Autodesk Fusion 360 part; units mm, degrees
(part 2 of 3)
sketch "Schizzo3 (7)" plane through (0, 0, 39.9) normal (0, 0, 1) x (1, 0, 0) in component "03A_Fermaglio_anti_sollevamento_Est_M3"
  line L0 (48.5, -5) -> (55, -5)
  line L1 (55, -5) -> (55, 5)
  line L2 (55, 5) -> (48.5, 5)
  line L3 (48.5, 5) -> (48.5, -5)
extrude "Estrusione_Linguetta_fermaglio_Est" add sketch "Schizzo3 (7)" along normal blind 3 bodies 8 in component "03A_Fermaglio_anti_sollevamento_Est_M3"
sketch "Schizzo4 (7)" plane through (0, 0, 33) normal (0, 0, 1) x (1, 0, 0) in component "03A_Fermaglio_anti_sollevamento_Est_M3"
  circle A0 centre (58.5, 0) radius 1.6
extrude "Foro_M3_fermaglio_Est" cut sketch "Schizzo4 (7)" along normal blind 3 bodies 8 in component "03A_Fermaglio_anti_sollevamento_Est_M3"
ref_plane "Piano di lavoro1" through (0, 0, 33) normal (0, 0, 1) x (1, 0, 0) in component "03A_Fermaglio_anti_sollevamento_Ovest_M3"
ref_plane "Piano di lavoro2" through (0, 0, 36) normal (0, 0, 1) x (1, 0, 0) in component "03A_Fermaglio_anti_sollevamento_Ovest_M3"
ref_plane "Piano di lavoro3" through (0, 0, 39.9) normal (0, 0, 1) x (1, 0, 0) in component "03A_Fermaglio_anti_sollevamento_Ovest_M3"
sketch "Schizzo1 (10)" plane through (0, 0, 33) normal (0, 0, 1) x (1, 0, 0) in component "03A_Fermaglio_anti_sollevamento_Ovest_M3"
  line L0 (-61.5, -5) -> (-51.5, -5)
  line L1 (-51.5, -5) -> (-51.5, 5)
  line L2 (-51.5, 5) -> (-61.5, 5)
  line L3 (-61.5, 5) -> (-61.5, -5)
extrude "Estrusione_Piede_fermaglio_Ovest" add sketch "Schizzo1 (10)" along normal blind 3 separate body makes body 9 in component "03A_Fermaglio_anti_sollevamento_Ovest_M3"
sketch "Schizzo2 (8)" plane through (0, 0, 36) normal (0, 0, 1) x (1, 0, 0) in component "03A_Fermaglio_anti_sollevamento_Ovest_M3"
  line L0 (-55, -5) -> (-52, -5)
  line L1 (-52, -5) -> (-52, 5)
  line L2 (-52, 5) -> (-55, 5)
  line L3 (-55, 5) -> (-55, -5)
extrude "Estrusione_Montante_fermaglio_Ovest" add sketch "Schizzo2 (8)" along normal blind 3.9 bodies 9 in component "03A_Fermaglio_anti_sollevamento_Ovest_M3"
sketch "Schizzo3 (8)" plane through (0, 0, 39.9) normal (0, 0, 1) x (1, 0, 0) in component "03A_Fermaglio_anti_sollevamento_Ovest_M3"
  line L0 (-55, -5) -> (-48.5, -5)
  line L1 (-48.5, -5) -> (-48.5, 5)
  line L2 (-48.5, 5) -> (-55, 5)
  line L3 (-55, 5) -> (-55, -5)
extrude "Estrusione_Linguetta_fermaglio_Ovest" add sketch "Schizzo3 (8)" along normal blind 3 bodies 9 in component "03A_Fermaglio_anti_sollevamento_Ovest_M3"
sketch "Schizzo4 (8)" plane through (0, 0, 33) normal (0, 0, 1) x (1, 0, 0) in component "03A_Fermaglio_anti_sollevamento_Ovest_M3"
  circle A0 centre (-58.5, 0) radius 1.6
extrude "Foro_M3_fermaglio_Ovest" cut sketch "Schizzo4 (8)" along normal blind 3 bodies 9 in component "03A_Fermaglio_anti_sollevamento_Ovest_M3"
ref_plane "Piano di lavoro1" through (0, 0, 33) normal (0, 0, 1) x (1, 0, 0) in component "03A_Fermaglio_anti_sollevamento_Nord_M3"
ref_plane "Piano di lavoro2" through (0, 0, 36) normal (0, 0, 1) x (1, 0, 0) in component "03A_Fermaglio_anti_sollevamento_Nord_M3"
ref_plane "Piano di lavoro3" through (0, 0, 39.9) normal (0, 0, 1) x (1, 0, 0) in component "03A_Fermaglio_anti_sollevamento_Nord_M3"
sketch "Schizzo1 (11)" plane through (0, 0, 33) normal (0, 0, 1) x (1, 0, 0) in component "03A_Fermaglio_anti_sollevamento_Nord_M3"
  line L0 (-5, 51.5) -> (5, 51.5)
  line L1 (5, 51.5) -> (5, 61.5)
  line L2 (5, 61.5) -> (-5, 61.5)
  line L3 (-5, 61.5) -> (-5, 51.5)
extrude "Estrusione_Piede_fermaglio_Nord" add sketch "Schizzo1 (11)" along normal blind 3 separate body makes body 10 in component "03A_Fermaglio_anti_sollevamento_Nord_M3"
sketch "Schizzo2 (9)" plane through (0, 0, 36) normal (0, 0, 1) x (1, 0, 0) in component "03A_Fermaglio_anti_sollevamento_Nord_M3"
  line L0 (-5, 52) -> (5, 52)
  line L1 (5, 52) -> (5, 55)
  line L2 (5, 55) -> (-5, 55)
  line L3 (-5, 55) -> (-5, 52)
extrude "Estrusione_Montante_fermaglio_Nord" add sketch "Schizzo2 (9)" along normal blind 3.9 bodies 10 in component "03A_Fermaglio_anti_sollevamento_Nord_M3"
sketch "Schizzo3 (9)" plane through (0, 0, 39.9) normal (0, 0, 1) x (1, 0, 0) in component "03A_Fermaglio_anti_sollevamento_Nord_M3"
  line L0 (-5, 48.5) -> (5, 48.5)
  line L1 (5, 48.5) -> (5, 55)
  line L2 (5, 55) -> (-5, 55)
  line L3 (-5, 55) -> (-5, 48.5)
extrude "Estrusione_Linguetta_fermaglio_Nord" add sketch "Schizzo3 (9)" along normal blind 3 bodies 10 in component "03A_Fermaglio_anti_sollevamento_Nord_M3"
sketch "Schizzo4 (9)" plane through (0, 0, 33) normal (0, 0, 1) x (1, 0, 0) in component "03A_Fermaglio_anti_sollevamento_Nord_M3"
  circle A0 centre (0, 58.5) radius 1.6
extrude "Foro_M3_fermaglio_Nord" cut sketch "Schizzo4 (9)" along normal blind 3 bodies 10 in component "03A_Fermaglio_anti_sollevamento_Nord_M3"
ref_plane "Piano di lavoro1" through (0, 0, 33) normal (0, 0, 1) x (1, 0, 0) in component "03A_Fermaglio_anti_sollevamento_Sud_M3"
ref_plane "Piano di lavoro2" through (0, 0, 36) normal (0, 0, 1) x (1, 0, 0) in component "03A_Fermaglio_anti_sollevamento_Sud_M3"
ref_plane "Piano di lavoro3" through (0, 0, 39.9) normal (0, 0, 1) x (1, 0, 0) in component "03A_Fermaglio_anti_sollevamento_Sud_M3"
sketch "Schizzo1 (12)" plane through (0, 0, 33) normal (0, 0, 1) x (1, 0, 0) in component "03A_Fermaglio_anti_sollevamento_Sud_M3"
  line L0 (-5, -61.5) -> (5, -61.5)
  line L1 (5, -61.5) -> (5, -51.5)
  line L2 (5, -51.5) -> (-5, -51.5)
  line L3 (-5, -51.5) -> (-5, -61.5)
extrude "Estrusione_Piede_fermaglio_Sud" add sketch "Schizzo1 (12)" along normal blind 3 separate body makes body 11 in component "03A_Fermaglio_anti_sollevamento_Sud_M3"
sketch "Schizzo2 (10)" plane through (0, 0, 36) normal (0, 0, 1) x (1, 0, 0) in component "03A_Fermaglio_anti_sollevamento_Sud_M3"
  line L0 (-5, -55) -> (5, -55)
  line L1 (5, -55) -> (5, -52)
  line L2 (5, -52) -> (-5, -52)
  line L3 (-5, -52) -> (-5, -55)
extrude "Estrusione_Montante_fermaglio_Sud" add sketch "Schizzo2 (10)" along normal blind 3.9 bodies 11 in component "03A_Fermaglio_anti_sollevamento_Sud_M3"
sketch "Schizzo3 (10)" plane through (0, 0, 39.9) normal (0, 0, 1) x (1, 0, 0) in component "03A_Fermaglio_anti_sollevamento_Sud_M3"
  line L0 (-5, -55) -> (5, -55)
  line L1 (5, -55) -> (5, -48.5)
  line L2 (5, -48.5) -> (-5, -48.5)
  line L3 (-5, -48.5) -> (-5, -55)
extrude "Estrusione_Linguetta_fermaglio_Sud" add sketch "Schizzo3 (10)" along normal blind 3 bodies 11 in component "03A_Fermaglio_anti_sollevamento_Sud_M3"
sketch "Schizzo4 (10)" plane through (0, 0, 33) normal (0, 0, 1) x (1, 0, 0) in component "03A_Fermaglio_anti_sollevamento_Sud_M3"
  circle A0 centre (0, -58.5) radius 1.6
extrude "Foro_M3_fermaglio_Sud" cut sketch "Schizzo4 (10)" along normal blind 3 bodies 11 in component "03A_Fermaglio_anti_sollevamento_Sud_M3"
ref_plane "Piano di lavoro1" through (0, 0, 45.5) normal (0, 0, 1) x (1, 0, 0) in component "04_Torretta_parte_fissa_azimut"
sketch "Schizzo1 (13)" plane through (0, 0, 45.5) normal (0, 0, 1) x (1, 0, 0) in component "04_Torretta_parte_fissa_azimut"
  line L0 (-40, -35) -> (40, -35)
  line L1 (40, -35) -> (40, 35)
  line L2 (40, 35) -> (-40, 35)
  line L3 (-40, 35) -> (-40, -35)
extrude "Estrusione_Base_parte_fissa" add sketch "Schizzo1 (13)" along normal blind 4 separate body makes body 12 in component "04_Torretta_parte_fissa_azimut"
ref_plane "Piano di lavoro2" through (0, 0, 39.5) normal (0, 0, 1) x (1, 0, 0) in component "04_Torretta_parte_fissa_azimut"
sketch "Schizzo2 (11)" plane through (0, 0, 39.5) normal (0, 0, 1) x (1, 0, 0) in component "04_Torretta_parte_fissa_azimut"
  circle A0 centre (-19, 0) radius 5
extrude "Estrusione_Distanziale_telaio_M3_01" add sketch "Schizzo2 (11)" along normal blind 6.2 bodies 12 in component "04_Torretta_parte_fissa_azimut"
sketch "Schizzo3 (11)" plane through (0, 0, 39.5) normal (0, 0, 1) x (1, 0, 0) in component "04_Torretta_parte_fissa_azimut"
  circle A0 centre (-19, 0) radius 1.6
extrude "Foro_M3_base_fissa_01" cut sketch "Schizzo3 (11)" along normal blind 10 bodies 12 in component "04_Torretta_parte_fissa_azimut"
sketch "Schizzo4 (11)" plane through (0, 0, 39.5) normal (0, 0, 1) x (1, 0, 0) in component "04_Torretta_parte_fissa_azimut"
  circle A0 centre (19, 0) radius 5
extrude "Estrusione_Distanziale_telaio_M3_02" add sketch "Schizzo4 (11)" along normal blind 6.2 bodies 12 in component "04_Torretta_parte_fissa_azimut"
sketch "Schizzo5 (6)" plane through (0, 0, 39.5) normal (0, 0, 1) x (1, 0, 0) in component "04_Torretta_parte_fissa_azimut"
  circle A0 centre (19, 0) radius 1.6
extrude "Foro_M3_base_fissa_02" cut sketch "Schizzo5 (6)" along normal blind 10 bodies 12 in component "04_Torretta_parte_fissa_azimut"
sketch "Schizzo6 (6)" plane through (0, 0, 39.5) normal (0, 0, 1) x (1, 0, 0) in component "04_Torretta_parte_fissa_azimut"
  circle A0 centre (0, -19) radius 5
extrude "Estrusione_Distanziale_telaio_M3_03" add sketch "Schizzo6 (6)" along normal blind 6.2 bodies 12 in component "04_Torretta_parte_fissa_azimut"
sketch "Schizzo7 (6)" plane through (0, 0, 39.5) normal (0, 0, 1) x (1, 0, 0) in component "04_Torretta_parte_fissa_azimut"
  circle A0 centre (0, -19) radius 1.6
extrude "Foro_M3_base_fissa_03" cut sketch "Schizzo7 (6)" along normal blind 10 bodies 12 in component "04_Torretta_parte_fissa_azimut"
sketch "Schizzo8 (6)" plane through (0, 0, 39.5) normal (0, 0, 1) x (1, 0, 0) in component "04_Torretta_parte_fissa_azimut"
  circle A0 centre (0, 19) radius 5
extrude "Estrusione_Distanziale_telaio_M3_04" add sketch "Schizzo8 (6)" along normal blind 6.2 bodies 12 in component "04_Torretta_parte_fissa_azimut"
sketch "Schizzo9 (6)" plane through (0, 0, 39.5) normal (0, 0, 1) x (1, 0, 0) in component "04_Torretta_parte_fissa_azimut"
  circle A0 centre (0, 19) radius 1.6
extrude "Foro_M3_base_fissa_04" cut sketch "Schizzo9 (6)" along normal blind 10 bodies 12 in component "04_Torretta_parte_fissa_azimut"
sketch "Schizzo10 (6)" plane through (0, 0, 45.5) normal (0, 0, 1) x (1, 0, 0) in component "04_Torretta_parte_fissa_azimut"
  line L0 (19.0919, 14.1421) -> (25.4558, 20.5061)
  line L1 (25.4558, 20.5061) -> (20.5061, 25.4558)
  line L2 (20.5061, 25.4558) -> (14.1421, 19.0919)
  line L3 (14.1421, 19.0919) -> (19.0919, 14.1421)
extrude "Passaggio_9x7_comune_servi_cannone_base_fissa" cut sketch "Schizzo10 (6)" along normal blind 4 bodies 12 in component "04_Torretta_parte_fissa_azimut"
sketch "Schizzo11 (6)" plane through (0, 0, 45.5) normal (0, 0, 1) x (1, 0, 0) in component "04_Torretta_parte_fissa_azimut"
  line L0 (-30.5, -19.5) -> (-25.5, -19.5)
  line L1 (-25.5, -19.5) -> (-25.5, -17.5)
  line L2 (-25.5, -17.5) -> (-30.5, -17.5)
  line L3 (-30.5, -17.5) -> (-30.5, -19.5)
extrude "Asola_fermacavo_Servo_sinistro_01" cut sketch "Schizzo11 (6)" along normal blind 4 bodies 12 in component "04_Torretta_parte_fissa_azimut"
sketch "Schizzo12 (5)" plane through (0, 0, 45.5) normal (0, 0, 1) x (1, 0, 0) in component "04_Torretta_parte_fissa_azimut"
  line L0 (-30.5, -12.5) -> (-25.5, -12.5)
  line L1 (-25.5, -12.5) -> (-25.5, -10.5)
  line L2 (-25.5, -10.5) -> (-30.5, -10.5)
  line L3 (-30.5, -10.5) -> (-30.5, -12.5)
extrude "Asola_fermacavo_Servo_sinistro_02" cut sketch "Schizzo12 (5)" along normal blind 4 bodies 12 in component "04_Torretta_parte_fissa_azimut"
sketch "Schizzo13 (5)" plane through (0, 0, 45.5) normal (0, 0, 1) x (1, 0, 0) in component "04_Torretta_parte_fissa_azimut"
  line L0 (-2.5, -11.5) -> (2.5, -11.5)
  line L1 (2.5, -11.5) -> (2.5, -9.5)
  line L2 (2.5, -9.5) -> (-2.5, -9.5)
  line L3 (-2.5, -9.5) -> (-2.5, -11.5)
extrude "Asola_fermacavo_Cannone_01" cut sketch "Schizzo13 (5)" along normal blind 4 bodies 12 in component "04_Torretta_parte_fissa_azimut"
sketch "Schizzo14 (4)" plane through (0, 0, 45.5) normal (0, 0, 1) x (1, 0, 0) in component "04_Torretta_parte_fissa_azimut"
  line L0 (-2.5, -4.5) -> (2.5, -4.5)
  line L1 (2.5, -4.5) -> (2.5, -2.5)
  line L2 (2.5, -2.5) -> (-2.5, -2.5)
  line L3 (-2.5, -2.5) -> (-2.5, -4.5)
extrude "Asola_fermacavo_Cannone_02" cut sketch "Schizzo14 (4)" along normal blind 4 bodies 12 in component "04_Torretta_parte_fissa_azimut"
sketch "Schizzo15 (4)" plane through (0, 0, 45.5) normal (0, 0, 1) x (1, 0, 0) in component "04_Torretta_parte_fissa_azimut"
  line L0 (25.5, -19.5) -> (30.5, -19.5)
  line L1 (30.5, -19.5) -> (30.5, -17.5)
  line L2 (30.5, -17.5) -> (25.5, -17.5)
  line L3 (25.5, -17.5) -> (25.5, -19.5)
extrude "Asola_fermacavo_Servo_destro_01" cut sketch "Schizzo15 (4)" along normal blind 4 bodies 12 in component "04_Torretta_parte_fissa_azimut"
sketch "Schizzo16 (4)" plane through (0, 0, 45.5) normal (0, 0, 1) x (1, 0, 0) in component "04_Torretta_parte_fissa_azimut"
  line L0 (25.5, -12.5) -> (30.5, -12.5)
  line L1 (30.5, -12.5) -> (30.5, -10.5)
  line L2 (30.5, -10.5) -> (25.5, -10.5)
  line L3 (25.5, -10.5) -> (25.5, -12.5)
extrude "Asola_fermacavo_Servo_destro_02" cut sketch "Schizzo16 (4)" along normal blind 4 bodies 12 in component "04_Torretta_parte_fissa_azimut"
ref_plane "Piano di lavoro3" through (-40, 0, 0) normal (1, 0, 0) x (0, 1, 0) in component "04_Torretta_parte_fissa_azimut"
sketch "Schizzo17 (4)" plane through (-40, 0, 0) normal (1, 0, 0) x (0, 0, -1) in component "04_Torretta_parte_fissa_azimut"
  line L0 (-49.5, -35) -> (-99.5, -35)
  line L1 (-99.5, -35) -> (-99.5, 35)
  line L2 (-99.5, 35) -> (-49.5, 35)
  line L3 (-49.5, 35) -> (-49.5, -35)
extrude "Estrusione_Parete_fissa_Sinistra" add sketch "Schizzo17 (4)" along normal blind 4 bodies 12 in component "04_Torretta_parte_fissa_azimut"
ref_plane "Piano di lavoro4" through (-40, 0, 0) normal (1, 0, 0) x (0, 1, 0) in component "04_Torretta_parte_fissa_azimut"
sketch "Schizzo18 (4)" plane through (-40, 0, 0) normal (1, 0, 0) x (0, 0, -1) in component "04_Torretta_parte_fissa_azimut"
  line L0 (-74.9, -17.5) -> (-88.1, -17.5)
  line L1 (-88.1, -17.5) -> (-88.1, 6.2)
  line L2 (-88.1, 6.2) -> (-74.9, 6.2)
  line L3 (-74.9, 6.2) -> (-74.9, -17.5)
extrude "Finestra_inserimento_SG90_Sinistra" cut sketch "Schizzo18 (4)" along normal blind 4 bodies 12 in component "04_Torretta_parte_fissa_azimut"
ref_plane "Piano di lavoro5" through (-40, 0, 0) normal (1, 0, 0) x (0, 1, 0) in component "04_Torretta_parte_fissa_azimut"
sketch "Schizzo19 (3)" plane through (-40, 0, 0) normal (1, 0, 0) x (0, 0, -1) in component "04_Torretta_parte_fissa_azimut"
  line L0 (-70.4, -8.15) -> (-74.9, -8.15)
  line L1 (-74.9, -8.15) -> (-74.9, -3.15)
  line L2 (-74.9, -3.15) -> (-70.4, -3.15)
  line L3 (-70.4, -3.15) -> (-70.4, -8.15)
extrude "Diramazione_cavo_5x4_5_SG90_Sinistra" cut sketch "Schizzo19 (3)" along normal blind 4 bodies 12 in component "04_Torretta_parte_fissa_azimut"
ref_plane "Piano di lavoro6" through (36, 0, 0) normal (1, 0, 0) x (0, 1, 0) in component "04_Torretta_parte_fissa_azimut"
sketch "Schizzo20 (3)" plane through (36, 0, 0) normal (1, 0, 0) x (0, 0, -1) in component "04_Torretta_parte_fissa_azimut"
  line L0 (-49.5, -35) -> (-99.5, -35)
  line L1 (-99.5, -35) -> (-99.5, 35)
  line L2 (-99.5, 35) -> (-49.5, 35)
  line L3 (-49.5, 35) -> (-49.5, -35)
extrude "Estrusione_Parete_fissa_Destra" add sketch "Schizzo20 (3)" along normal blind 4 bodies 12 in component "04_Torretta_parte_fissa_azimut"
ref_plane "Piano di lavoro7" through (36, 0, 0) normal (1, 0, 0) x (0, 1, 0) in component "04_Torretta_parte_fissa_azimut"
sketch "Schizzo21 (3)" plane through (36, 0, 0) normal (1, 0, 0) x (0, 0, -1) in component "04_Torretta_parte_fissa_azimut"
  line L0 (-74.9, -17.5) -> (-88.1, -17.5)
  line L1 (-88.1, -17.5) -> (-88.1, 6.2)
  line L2 (-88.1, 6.2) -> (-74.9, 6.2)
  line L3 (-74.9, 6.2) -> (-74.9, -17.5)
extrude "Finestra_inserimento_SG90_Destra" cut sketch "Schizzo21 (3)" along normal blind 4 bodies 12 in component "04_Torretta_parte_fissa_azimut"
ref_plane "Piano di lavoro8" through (36, 0, 0) normal (1, 0, 0) x (0, 1, 0) in component "04_Torretta_parte_fissa_azimut"
sketch "Schizzo22 (3)" plane through (36, 0, 0) normal (1, 0, 0) x (0, 0, -1) in component "04_Torretta_parte_fissa_azimut"
  line L0 (-70.4, -8.15) -> (-74.9, -8.15)
  line L1 (-74.9, -8.15) -> (-74.9, -3.15)
  line L2 (-74.9, -3.15) -> (-70.4, -3.15)
  line L3 (-70.4, -3.15) -> (-70.4, -8.15)
extrude "Diramazione_cavo_5x4_5_SG90_Destra" cut sketch "Schizzo22 (3)" along normal blind 4 bodies 12 in component "04_Torretta_parte_fissa_azimut"
ref_plane "Piano di lavoro9" through (0, 0, 72.4) normal (0, 0, 1) x (1, 0, 0) in component "04_Torretta_parte_fissa_azimut"
sketch "Schizzo23 (2)" plane through (0, 0, 72.4) normal (0, 0, 1) x (1, 0, 0) in component "04_Torretta_parte_fissa_azimut"
  line L0 (-63.5, -24.8) -> (-40, -24.8)
  line L1 (-40, -24.8) -> (-40, 13.5)
  line L2 (-40, 13.5) -> (-63.5, 13.5)
  line L3 (-63.5, 13.5) -> (-63.5, -24.8)
extrude "Estrusione_Slitta_SG90_Sinistra_ripiano_Inferiore" add sketch "Schizzo23 (2)" along normal blind 2.5 bodies 12 in component "04_Torretta_parte_fissa_azimut"
ref_plane "Piano di lavoro10" through (0, 0, 88.1) normal (0, 0, 1) x (1, 0, 0) in component "04_Torretta_parte_fissa_azimut"
sketch "Schizzo24 (2)" plane through (0, 0, 88.1) normal (0, 0, 1) x (1, 0, 0) in component "04_Torretta_parte_fissa_azimut"
  line L0 (-63.5, -24.8) -> (-40, -24.8)
  line L1 (-40, -24.8) -> (-40, 13.5)
  line L2 (-40, 13.5) -> (-63.5, 13.5)
  line L3 (-63.5, 13.5) -> (-63.5, -24.8)
extrude "Estrusione_Slitta_SG90_Sinistra_ripiano_Superiore" add sketch "Schizzo24 (2)" along normal blind 2.5 bodies 12 in component "04_Torretta_parte_fissa_azimut"
ref_plane "Piano di lavoro11" through (0, 0, 72.4) normal (0, 0, 1) x (1, 0, 0) in component "04_Torretta_parte_fissa_azimut"
sketch "Schizzo25 (2)" plane through (0, 0, 72.4) normal (0, 0, 1) x (1, 0, 0) in component "04_Torretta_parte_fissa_azimut"
  line L0 (-63.5, -8.15) -> (-61.5, -8.15)
  line L1 (-61.5, -8.15) -> (-61.5, -3.15)
  line L2 (-61.5, -3.15) -> (-63.5, -3.15)
  line L3 (-63.5, -3.15) -> (-63.5, -8.15)
extrude "Uscita_cavo_5x2_SG90_Sinistra" cut sketch "Schizzo25 (2)" along normal blind 2.5 bodies 12 in component "04_Torretta_parte_fissa_azimut"
ref_plane "Piano di lavoro12" through (-63.5, 0, 0) normal (1, 0, 0) x (0, 1, 0) in component "04_Torretta_parte_fissa_azimut"
sketch "Schizzo26 (2)" plane through (-63.5, 0, 0) normal (1, 0, 0) x (0, 0, -1) in component "04_Torretta_parte_fissa_azimut"
  line L0 (-74.9, -24.8) -> (-88.1, -24.8)
  line L1 (-88.1, -24.8) -> (-88.1, -22.3)
  line L2 (-88.1, -22.3) -> (-74.9, -22.3)
  line L3 (-74.9, -22.3) -> (-74.9, -24.8)
extrude "Estrusione_Slitta_SG90_Sinistra_guida_01" add sketch "Schizzo26 (2)" along normal blind 23.5 bodies 12 in component "04_Torretta_parte_fissa_azimut"
ref_plane "Piano di lavoro13" through (-63.5, 0, 0) normal (1, 0, 0) x (0, 1, 0) in component "04_Torretta_parte_fissa_azimut"
sketch "Schizzo27 (2)" plane through (-63.5, 0, 0) normal (1, 0, 0) x (0, 0, -1) in component "04_Torretta_parte_fissa_azimut"
  line L0 (-74.9, 11) -> (-88.1, 11)
  line L1 (-88.1, 11) -> (-88.1, 13.5)
  line L2 (-88.1, 13.5) -> (-74.9, 13.5)
  line L3 (-74.9, 13.5) -> (-74.9, 11)
extrude "Estrusione_Slitta_SG90_Sinistra_guida_02" add sketch "Schizzo27 (2)" along normal blind 23.5 bodies 12 in component "04_Torretta_parte_fissa_azimut"
ref_plane "Piano di lavoro14" through (-63.5, 0, 0) normal (1, 0, 0) x (0, 1, 0) in component "04_Torretta_parte_fissa_azimut"
sketch "Schizzo28 (2)" plane through (-63.5, 0, 0) normal (1, 0, 0) x (0, 0, -1) in component "04_Torretta_parte_fissa_azimut"
  circle A0 centre (-81.5, -23.55) radius 1.1
extrude "Preforo_M2_5_slitta_Sinistra_01" cut sketch "Schizzo28 (2)" along normal blind 23.5 bodies 12 in component "04_Torretta_parte_fissa_azimut"
ref_plane "Piano di lavoro15" through (-63.5, 0, 0) normal (1, 0, 0) x (0, 1, 0) in component "04_Torretta_parte_fissa_azimut"
sketch "Schizzo29 (2)" plane through (-63.5, 0, 0) normal (1, 0, 0) x (0, 0, -1) in component "04_Torretta_parte_fissa_azimut"
  circle A0 centre (-81.5, 12.25) radius 1.1
extrude "Preforo_M2_5_slitta_Sinistra_02" cut sketch "Schizzo29 (2)" along normal blind 23.5 bodies 12 in component "04_Torretta_parte_fissa_azimut"
ref_plane "Piano di lavoro16" through (0, 0, 72.4) normal (0, 0, 1) x (1, 0, 0) in component "04_Torretta_parte_fissa_azimut"
sketch "Schizzo30 (2)" plane through (0, 0, 72.4) normal (0, 0, 1) x (1, 0, 0) in component "04_Torretta_parte_fissa_azimut"
  line L0 (40, -24.8) -> (63.5, -24.8)
  line L1 (63.5, -24.8) -> (63.5, 13.5)
  line L2 (63.5, 13.5) -> (40, 13.5)
  line L3 (40, 13.5) -> (40, -24.8)
extrude "Estrusione_Slitta_SG90_Destra_ripiano_Inferiore" add sketch "Schizzo30 (2)" along normal blind 2.5 bodies 12 in component "04_Torretta_parte_fissa_azimut"
ref_plane "Piano di lavoro17" through (0, 0, 88.1) normal (0, 0, 1) x (1, 0, 0) in component "04_Torretta_parte_fissa_azimut"
sketch "Schizzo31 (2)" plane through (0, 0, 88.1) normal (0, 0, 1) x (1, 0, 0) in component "04_Torretta_parte_fissa_azimut"
  line L0 (40, -24.8) -> (63.5, -24.8)
  line L1 (63.5, -24.8) -> (63.5, 13.5)
  line L2 (63.5, 13.5) -> (40, 13.5)
  line L3 (40, 13.5) -> (40, -24.8)
extrude "Estrusione_Slitta_SG90_Destra_ripiano_Superiore" add sketch "Schizzo31 (2)" along normal blind 2.5 bodies 12 in component "04_Torretta_parte_fissa_azimut"
ref_plane "Piano di lavoro18" through (0, 0, 72.4) normal (0, 0, 1) x (1, 0, 0) in component "04_Torretta_parte_fissa_azimut"
sketch "Schizzo32 (2)" plane through (0, 0, 72.4) normal (0, 0, 1) x (1, 0, 0) in component "04_Torretta_parte_fissa_azimut"
  line L0 (61.5, -8.15) -> (63.5, -8.15)
  line L1 (63.5, -8.15) -> (63.5, -3.15)
  line L2 (63.5, -3.15) -> (61.5, -3.15)
  line L3 (61.5, -3.15) -> (61.5, -8.15)
extrude "Uscita_cavo_5x2_SG90_Destra" cut sketch "Schizzo32 (2)" along normal blind 2.5 bodies 12 in component "04_Torretta_parte_fissa_azimut"
ref_plane "Piano di lavoro19" through (40, 0, 0) normal (1, 0, 0) x (0, 1, 0) in component "04_Torretta_parte_fissa_azimut"
sketch "Schizzo33 (2)" plane through (40, 0, 0) normal (1, 0, 0) x (0, 0, -1) in component "04_Torretta_parte_fissa_azimut"
  line L0 (-74.9, -24.8) -> (-88.1, -24.8)
  line L1 (-88.1, -24.8) -> (-88.1, -22.3)
  line L2 (-88.1, -22.3) -> (-74.9, -22.3)
  line L3 (-74.9, -22.3) -> (-74.9, -24.8)
extrude "Estrusione_Slitta_SG90_Destra_guida_01" add sketch "Schizzo33 (2)" along normal blind 23.5 bodies 12 in component "04_Torretta_parte_fissa_azimut"
ref_plane "Piano di lavoro20" through (40, 0, 0) normal (1, 0, 0) x (0, 1, 0) in component "04_Torretta_parte_fissa_azimut"
sketch "Schizzo34 (2)" plane through (40, 0, 0) normal (1, 0, 0) x (0, 0, -1) in component "04_Torretta_parte_fissa_azimut"
  line L0 (-74.9, 11) -> (-88.1, 11)
  line L1 (-88.1, 11) -> (-88.1, 13.5)
  line L2 (-88.1, 13.5) -> (-74.9, 13.5)
  line L3 (-74.9, 13.5) -> (-74.9, 11)
extrude "Estrusione_Slitta_SG90_Destra_guida_02" add sketch "Schizzo34 (2)" along normal blind 23.5 bodies 12 in component "04_Torretta_parte_fissa_azimut"
ref_plane "Piano di lavoro21" through (40, 0, 0) normal (1, 0, 0) x (0, 1, 0) in component "04_Torretta_parte_fissa_azimut"
sketch "Schizzo35 (2)" plane through (40, 0, 0) normal (1, 0, 0) x (0, 0, -1) in component "04_Torretta_parte_fissa_azimut"
  circle A0 centre (-81.5, -23.55) radius 1.1
extrude "Preforo_M2_5_slitta_Destra_01" cut sketch "Schizzo35 (2)" along normal blind 23.5 bodies 12 in component "04_Torretta_parte_fissa_azimut"
ref_plane "Piano di lavoro22" through (40, 0, 0) normal (1, 0, 0) x (0, 1, 0) in component "04_Torretta_parte_fissa_azimut"
sketch "Schizzo36 (2)" plane through (40, 0, 0) normal (1, 0, 0) x (0, 0, -1) in component "04_Torretta_parte_fissa_azimut"
  circle A0 centre (-81.5, 12.25) radius 1.1
extrude "Preforo_M2_5_slitta_Destra_02" cut sketch "Schizzo36 (2)" along normal blind 23.5 bodies 12 in component "04_Torretta_parte_fissa_azimut"
ref_plane "Piano di lavoro1" through (-63, 0, 0) normal (1, 0, 0) x (0, 1, 0) in component "05_Servo_TowerPro_SG90_Sinistro_riferimento"
sketch "Schizzo1 (14)" plane through (-63, 0, 0) normal (1, 0, 0) x (0, 0, -1) in component "05_Servo_TowerPro_SG90_Sinistro_riferimento"
  line L0 (-75.4, -17) -> (-87.6, -17)
  line L1 (-87.6, -17) -> (-87.6, 5.7)
  line L2 (-87.6, 5.7) -> (-75.4, 5.7)
  line L3 (-75.4, 5.7) -> (-75.4, -17)
extrude "Estrusione_Corpo_SG90_Sinistro" add sketch "Schizzo1 (14)" along normal blind 27 separate body makes body 13 in component "05_Servo_TowerPro_SG90_Sinistro_riferimento"
ref_plane "Piano di lavoro2" through (-36, 0, 0) normal (1, 0, 0) x (0, 1, 0) in component "05_Servo_TowerPro_SG90_Sinistro_riferimento"
sketch "Schizzo2 (12)" plane through (-36, 0, 0) normal (1, 0, 0) x (0, 0, -1) in component "05_Servo_TowerPro_SG90_Sinistro_riferimento"
  circle A0 centre (-81.5, 0) radius 3
extrude "Estrusione_Albero_uscita_SG90_Sinistro" add sketch "Schizzo2 (12)" along normal blind 3.3 bodies 13 in component "05_Servo_TowerPro_SG90_Sinistro_riferimento"
ref_plane "Piano di lavoro1" through (36, 0, 0) normal (1, 0, 0) x (0, 1, 0) in component "06_Servo_TowerPro_SG90_Destro_riferimento"
sketch "Schizzo1 (15)" plane through (36, 0, 0) normal (1, 0, 0) x (0, 0, -1) in component "06_Servo_TowerPro_SG90_Destro_riferimento"
  line L0 (-75.4, -17) -> (-87.6, -17)
  line L1 (-87.6, -17) -> (-87.6, 5.7)
  line L2 (-87.6, 5.7) -> (-75.4, 5.7)
  line L3 (-75.4, 5.7) -> (-75.4, -17)
extrude "Estrusione_Corpo_SG90_Destro" add sketch "Schizzo1 (15)" along normal blind 27 separate body makes body 14 in component "06_Servo_TowerPro_SG90_Destro_riferimento"
ref_plane "Piano di lavoro2" through (32.7, 0, 0) normal (1, 0, 0) x (0, 1, 0) in component "06_Servo_TowerPro_SG90_Destro_riferimento"
sketch "Schizzo2 (13)" plane through (32.7, 0, 0) normal (1, 0, 0) x (0, 0, -1) in component "06_Servo_TowerPro_SG90_Destro_riferimento"
  circle A0 centre (-81.5, 0) radius 3
extrude "Estrusione_Albero_uscita_SG90_Destro" add sketch "Schizzo2 (13)" along normal blind 3.3 bodies 14 in component "06_Servo_TowerPro_SG90_Destro_riferimento"
ref_plane "Piano di lavoro1" through (-66.5, 0, 0) normal (1, 0, 0) x (0, 1, 0) in component "07_Barrette_removibili_M2_5_SG90_Sinistra"
sketch "Schizzo1 (16)" plane through (-66.5, 0, 0) normal (1, 0, 0) x (0, 0, -1) in component "07_Barrette_removibili_M2_5_SG90_Sinistra"
  line L0 (-74.9, -24.8) -> (-88.1, -24.8)
  line L1 (-88.1, -24.8) -> (-88.1, -14)
  line L2 (-88.1, -14) -> (-74.9, -14)
  line L3 (-74.9, -14) -> (-74.9, -24.8)
extrude "Estrusione_Barretta_Sinistra_01" add sketch "Schizzo1 (16)" along normal blind 3 separate body makes body 15 in component "07_Barrette_removibili_M2_5_SG90_Sinistra"
ref_plane "Piano di lavoro2" through (-66.5, 0, 0) normal (1, 0, 0) x (0, 1, 0) in component "07_Barrette_removibili_M2_5_SG90_Sinistra"
sketch "Schizzo2 (14)" plane through (-66.5, 0, 0) normal (1, 0, 0) x (0, 0, -1) in component "07_Barrette_removibili_M2_5_SG90_Sinistra"
  circle A0 centre (-81.5, -23.55) radius 1.35
extrude "Foro_M2_5_barretta_Sinistra_01" cut sketch "Schizzo2 (14)" along normal blind 3 bodies 15 in component "07_Barrette_removibili_M2_5_SG90_Sinistra"
ref_plane "Piano di lavoro3" through (-66.5, 0, 0) normal (1, 0, 0) x (0, 1, 0) in component "07_Barrette_removibili_M2_5_SG90_Sinistra"
sketch "Schizzo3 (12)" plane through (-66.5, 0, 0) normal (1, 0, 0) x (0, 0, -1) in component "07_Barrette_removibili_M2_5_SG90_Sinistra"
  line L0 (-74.9, 2.7) -> (-88.1, 2.7)
  line L1 (-88.1, 2.7) -> (-88.1, 13.5)
  line L2 (-88.1, 13.5) -> (-74.9, 13.5)
  line L3 (-74.9, 13.5) -> (-74.9, 2.7)
extrude "Estrusione_Barretta_Sinistra_02" add sketch "Schizzo3 (12)" along normal blind 3 separate body makes body 16 in component "07_Barrette_removibili_M2_5_SG90_Sinistra"
ref_plane "Piano di lavoro4" through (-66.5, 0, 0) normal (1, 0, 0) x (0, 1, 0) in component "07_Barrette_removibili_M2_5_SG90_Sinistra"
sketch "Schizzo4 (12)" plane through (-66.5, 0, 0) normal (1, 0, 0) x (0, 0, -1) in component "07_Barrette_removibili_M2_5_SG90_Sinistra"
  circle A0 centre (-81.5, 12.25) radius 1.35
extrude "Foro_M2_5_barretta_Sinistra_02" cut sketch "Schizzo4 (12)" along normal blind 3 bodies 16 in component "07_Barrette_removibili_M2_5_SG90_Sinistra"
ref_plane "Piano di lavoro1" through (63.5, 0, 0) normal (1, 0, 0) x (0, 1, 0) in component "08_Barrette_removibili_M2_5_SG90_Destra"
sketch "Schizzo1 (17)" plane through (63.5, 0, 0) normal (1, 0, 0) x (0, 0, -1) in component "08_Barrette_removibili_M2_5_SG90_Destra"
  line L0 (-74.9, -24.8) -> (-88.1, -24.8)
  line L1 (-88.1, -24.8) -> (-88.1, -14)
  line L2 (-88.1, -14) -> (-74.9, -14)
  line L3 (-74.9, -14) -> (-74.9, -24.8)
extrude "Estrusione_Barretta_Destra_01" add sketch "Schizzo1 (17)" along normal blind 3 separate body makes body 17 in component "08_Barrette_removibili_M2_5_SG90_Destra"
ref_plane "Piano di lavoro2" through (63.5, 0, 0) normal (1, 0, 0) x (0, 1, 0) in component "08_Barrette_removibili_M2_5_SG90_Destra"
sketch "Schizzo2 (15)" plane through (63.5, 0, 0) normal (1, 0, 0) x (0, 0, -1) in component "08_Barrette_removibili_M2_5_SG90_Destra"
  circle A0 centre (-81.5, -23.55) radius 1.35
extrude "Foro_M2_5_barretta_Destra_01" cut sketch "Schizzo2 (15)" along normal blind 3 bodies 17 in component "08_Barrette_removibili_M2_5_SG90_Destra"
ref_plane "Piano di lavoro3" through (63.5, 0, 0) normal (1, 0, 0) x (0, 1, 0) in component "08_Barrette_removibili_M2_5_SG90_Destra"
sketch "Schizzo3 (13)" plane through (63.5, 0, 0) normal (1, 0, 0) x (0, 0, -1) in component "08_Barrette_removibili_M2_5_SG90_Destra"
  line L0 (-74.9, 2.7) -> (-88.1, 2.7)
  line L1 (-88.1, 2.7) -> (-88.1, 13.5)
  line L2 (-88.1, 13.5) -> (-74.9, 13.5)
  line L3 (-74.9, 13.5) -> (-74.9, 2.7)
extrude "Estrusione_Barretta_Destra_02" add sketch "Schizzo3 (13)" along normal blind 3 separate body makes body 18 in component "08_Barrette_removibili_M2_5_SG90_Destra"
ref_plane "Piano di lavoro4" through (63.5, 0, 0) normal (1, 0, 0) x (0, 1, 0) in component "08_Barrette_removibili_M2_5_SG90_Destra"
sketch "Schizzo4 (13)" plane through (63.5, 0, 0) normal (1, 0, 0) x (0, 0, -1) in component "08_Barrette_removibili_M2_5_SG90_Destra"
  circle A0 centre (-81.5, 12.25) radius 1.35
extrude "Foro_M2_5_barretta_Destra_02" cut sketch "Schizzo4 (13)" along normal blind 3 bodies 18 in component "08_Barrette_removibili_M2_5_SG90_Destra"
ref_plane "Piano di lavoro1" through (0, 0, 79.5) normal (0, 0, 1) x (1, 0, 0) in component "09_Torretta_parte_mobile_elevazione"
sketch "Schizzo1 (18)" plane through (0, 0, 79.5) normal (0, 0, 1) x (1, 0, 0) in component "09_Torretta_parte_mobile_elevazione"
  line L0 (-34, -20) -> (34, -20)
  line L1 (34, -20) -> (34, 50)
  line L2 (34, 50) -> (-34, 50)
  line L3 (-34, 50) -> (-34, -20)
extrude "Estrusione_Piastra_culla_mobile" add sketch "Schizzo1 (18)" along normal blind 4 separate body makes body 19 in component "09_Torretta_parte_mobile_elevazione"
sketch "Schizzo2 (16)" plane through (0, 0, 79.5) normal (0, 0, 1) x (1, 0, 0) in component "09_Torretta_parte_mobile_elevazione"
  line L0 (-3, -17) -> (3, -17)
  line L1 (3, -17) -> (3, -13)
  line L2 (3, -13) -> (-3, -13)
  line L3 (-3, -13) -> (-3, -17)
extrude "Passaggio_6x4_connettore_cannone_sotto_culla" cut sketch "Schizzo2 (16)" along normal blind 4 bodies 19 in component "09_Torretta_parte_mobile_elevazione"
sketch "Schizzo3 (14)" plane through (0, 0, 79.5) normal (0, 0, 1) x (1, 0, 0) in component "09_Torretta_parte_mobile_elevazione"
  line L0 (-7, -17.5) -> (-5, -17.5)
  line L1 (-5, -17.5) -> (-5, -12.5)
  line L2 (-5, -12.5) -> (-7, -12.5)
  line L3 (-7, -12.5) -> (-7, -17.5)
extrude "Asola_fascetta_ansa_cannone_mobile_01" cut sketch "Schizzo3 (14)" along normal blind 4 bodies 19 in component "09_Torretta_parte_mobile_elevazione"
sketch "Schizzo4 (14)" plane through (0, 0, 79.5) normal (0, 0, 1) x (1, 0, 0) in component "09_Torretta_parte_mobile_elevazione"
  line L0 (5, -17.5) -> (7, -17.5)
  line L1 (7, -17.5) -> (7, -12.5)
  line L2 (7, -12.5) -> (5, -12.5)
  line L3 (5, -12.5) -> (5, -17.5)
extrude "Asola_fascetta_ansa_cannone_mobile_02" cut sketch "Schizzo4 (14)" along normal blind 4 bodies 19 in component "09_Torretta_parte_mobile_elevazione"
sketch "Schizzo5 (7)" plane through (0, 0, 79.5) normal (0, 0, 1) x (1, 0, 0) in component "09_Torretta_parte_mobile_elevazione"
  circle A0 centre (-20, -5) radius 1.75
extrude "Foro_fissaggio_PCB_cannone_01" cut sketch "Schizzo5 (7)" along normal blind 4 bodies 19 in component "09_Torretta_parte_mobile_elevazione"
sketch "Schizzo6 (7)" plane through (0, 0, 79.5) normal (0, 0, 1) x (1, 0, 0) in component "09_Torretta_parte_mobile_elevazione"
  line L0 (-17.1, -3.3257) -> (-20, -1.6514)
  line L1 (-20, -1.6514) -> (-22.9, -3.3257)
  line L2 (-22.9, -3.3257) -> (-22.9, -6.6743)
  line L3 (-22.9, -6.6743) -> (-20, -8.3486)
  line L4 (-20, -8.3486) -> (-17.1, -6.6743)
  line L5 (-17.1, -6.6743) -> (-17.1, -3.3257)
extrude "Sede_dado_M3_PCB_cannone_01" cut sketch "Schizzo6 (7)" along normal blind 2.6 bodies 19 in component "09_Torretta_parte_mobile_elevazione"
sketch "Schizzo7 (7)" plane through (0, 0, 79.5) normal (0, 0, 1) x (1, 0, 0) in component "09_Torretta_parte_mobile_elevazione"
  circle A0 centre (20, -5) radius 1.75
extrude "Foro_fissaggio_PCB_cannone_02" cut sketch "Schizzo7 (7)" along normal blind 4 bodies 19 in component "09_Torretta_parte_mobile_elevazione"
sketch "Schizzo8 (7)" plane through (0, 0, 79.5) normal (0, 0, 1) x (1, 0, 0) in component "09_Torretta_parte_mobile_elevazione"
  line L0 (22.9, -3.3257) -> (20, -1.6514)
  line L1 (20, -1.6514) -> (17.1, -3.3257)
  line L2 (17.1, -3.3257) -> (17.1, -6.6743)
  line L3 (17.1, -6.6743) -> (20, -8.3486)
  line L4 (20, -8.3486) -> (22.9, -6.6743)
  line L5 (22.9, -6.6743) -> (22.9, -3.3257)
extrude "Sede_dado_M3_PCB_cannone_02" cut sketch "Schizzo8 (7)" along normal blind 2.6 bodies 19 in component "09_Torretta_parte_mobile_elevazione"
sketch "Schizzo9 (7)" plane through (0, 0, 79.5) normal (0, 0, 1) x (1, 0, 0) in component "09_Torretta_parte_mobile_elevazione"
  circle A0 centre (-20, 35) radius 1.75
extrude "Foro_fissaggio_PCB_cannone_03" cut sketch "Schizzo9 (7)" along normal blind 4 bodies 19 in component "09_Torretta_parte_mobile_elevazione"
sketch "Schizzo10 (7)" plane through (0, 0, 79.5) normal (0, 0, 1) x (1, 0, 0) in component "09_Torretta_parte_mobile_elevazione"
  line L0 (-17.1, 36.6743) -> (-20, 38.3486)
  line L1 (-20, 38.3486) -> (-22.9, 36.6743)
  line L2 (-22.9, 36.6743) -> (-22.9, 33.3257)
  line L3 (-22.9, 33.3257) -> (-20, 31.6514)
  line L4 (-20, 31.6514) -> (-17.1, 33.3257)
  line L5 (-17.1, 33.3257) -> (-17.1, 36.6743)
extrude "Sede_dado_M3_PCB_cannone_03" cut sketch "Schizzo10 (7)" along normal blind 2.6 bodies 19 in component "09_Torretta_parte_mobile_elevazione"
sketch "Schizzo11 (7)" plane through (0, 0, 79.5) normal (0, 0, 1) x (1, 0, 0) in component "09_Torretta_parte_mobile_elevazione"
  circle A0 centre (20, 35) radius 1.75
extrude "Foro_fissaggio_PCB_cannone_04" cut sketch "Schizzo11 (7)" along normal blind 4 bodies 19 in component "09_Torretta_parte_mobile_elevazione"
sketch "Schizzo12 (6)" plane through (0, 0, 79.5) normal (0, 0, 1) x (1, 0, 0) in component "09_Torretta_parte_mobile_elevazione"
  line L0 (22.9, 36.6743) -> (20, 38.3486)
  line L1 (20, 38.3486) -> (17.1, 36.6743)
  line L2 (17.1, 36.6743) -> (17.1, 33.3257)
  line L3 (17.1, 33.3257) -> (20, 31.6514)
  line L4 (20, 31.6514) -> (22.9, 33.3257)
  line L5 (22.9, 33.3257) -> (22.9, 36.6743)
extrude "Sede_dado_M3_PCB_cannone_04" cut sketch "Schizzo12 (6)" along normal blind 2.6 bodies 19 in component "09_Torretta_parte_mobile_elevazione"
ref_plane "Piano di lavoro2" through (-34, 0, 0) normal (1, 0, 0) x (0, 1, 0) in component "09_Torretta_parte_mobile_elevazione"
sketch "Schizzo13 (6)" plane through (-34, 0, 0) normal (1, 0, 0) x (0, 0, -1) in component "09_Torretta_parte_mobile_elevazione"
  line L0 (-70.5, -12) -> (-92.5, -12)
  line L1 (-92.5, -12) -> (-92.5, 12)
  line L2 (-92.5, 12) -> (-70.5, 12)
  line L3 (-70.5, 12) -> (-70.5, -12)
extrude "Estrusione_Orecchio_mobile_Sinistra" add sketch "Schizzo13 (6)" along normal blind 4 bodies 19 in component "09_Torretta_parte_mobile_elevazione"
ref_plane "Piano di lavoro3" through (30, 0, 0) normal (1, 0, 0) x (0, 1, 0) in component "09_Torretta_parte_mobile_elevazione"
sketch "Schizzo14 (5)" plane through (30, 0, 0) normal (1, 0, 0) x (0, 0, -1) in component "09_Torretta_parte_mobile_elevazione"
  line L0 (-70.5, -12) -> (-92.5, -12)
  line L1 (-92.5, -12) -> (-92.5, 12)
  line L2 (-92.5, 12) -> (-70.5, 12)
  line L3 (-70.5, 12) -> (-70.5, -12)
extrude "Estrusione_Orecchio_mobile_Destra" add sketch "Schizzo14 (5)" along normal blind 4 bodies 19 in component "09_Torretta_parte_mobile_elevazione"
ref_plane "Piano di lavoro4" through (-40, 0, 0) normal (1, 0, 0) x (0, 1, 0) in component "09_Torretta_parte_mobile_elevazione"
sketch "Schizzo15 (5)" plane through (-40, 0, 0) normal (1, 0, 0) x (0, 0, -1) in component "09_Torretta_parte_mobile_elevazione"
  circle A0 centre (-81.5, 0) radius 3
extrude "Estrusione_Perno_servo_sinistro_coassiale" add sketch "Schizzo15 (5)" along normal blind 10 bodies 19 in component "09_Torretta_parte_mobile_elevazione"
ref_plane "Piano di lavoro5" through (30, 0, 0) normal (1, 0, 0) x (0, 1, 0) in component "09_Torretta_parte_mobile_elevazione"
sketch "Schizzo16 (5)" plane through (30, 0, 0) normal (1, 0, 0) x (0, 0, -1) in component "09_Torretta_parte_mobile_elevazione"
  circle A0 centre (-81.5, 0) radius 3
extrude "Estrusione_Perno_servo_destro_coassiale" add sketch "Schizzo16 (5)" along normal blind 10 bodies 19 in component "09_Torretta_parte_mobile_elevazione"
ref_plane "Piano di lavoro1" through (0, 0, 83.5) normal (0, 0, 1) x (1, 0, 0) in component "10_Modulo_cannone_reale_PCB_solenoide_canna"
sketch "Schizzo1 (19)" plane through (0, 0, 83.5) normal (0, 0, 1) x (1, 0, 0) in component "10_Modulo_cannone_reale_PCB_solenoide_canna"
  line L0 (-25, -10) -> (25, -10)
  line L1 (25, -10) -> (25, 40)
  line L2 (25, 40) -> (-25, 40)
  line L3 (-25, 40) -> (-25, -10)
extrude "Estrusione_PCB_modulo_cannone_50x50" add sketch "Schizzo1 (19)" along normal blind 2 separate body makes body 20 in component "10_Modulo_cannone_reale_PCB_solenoide_canna"
sketch "Schizzo2 (17)" plane through (0, 0, 83.5) normal (0, 0, 1) x (1, 0, 0) in component "10_Modulo_cannone_reale_PCB_solenoide_canna"
  circle A0 centre (-20, -5) radius 1.75
extrude "Foro_PCB_reale_01" cut sketch "Schizzo2 (17)" along normal blind 2 bodies 20 in component "10_Modulo_cannone_reale_PCB_solenoide_canna"
sketch "Schizzo3 (15)" plane through (0, 0, 83.5) normal (0, 0, 1) x (1, 0, 0) in component "10_Modulo_cannone_reale_PCB_solenoide_canna"
  circle A0 centre (20, -5) radius 1.75
extrude "Foro_PCB_reale_02" cut sketch "Schizzo3 (15)" along normal blind 2 bodies 20 in component "10_Modulo_cannone_reale_PCB_solenoide_canna"
sketch "Schizzo4 (15)" plane through (0, 0, 83.5) normal (0, 0, 1) x (1, 0, 0) in component "10_Modulo_cannone_reale_PCB_solenoide_canna"
  circle A0 centre (-20, 35) radius 1.75
extrude "Foro_PCB_reale_03" cut sketch "Schizzo4 (15)" along normal blind 2 bodies 20 in component "10_Modulo_cannone_reale_PCB_solenoide_canna"
sketch "Schizzo5 (8)" plane through (0, 0, 83.5) normal (0, 0, 1) x (1, 0, 0) in component "10_Modulo_cannone_reale_PCB_solenoide_canna"
  circle A0 centre (20, 35) radius 1.75
extrude "Foro_PCB_reale_04" cut sketch "Schizzo5 (8)" along normal blind 2 bodies 20 in component "10_Modulo_cannone_reale_PCB_solenoide_canna"
ref_plane "Piano di lavoro2" through (0, 0, 85.5) normal (0, 0, 1) x (1, 0, 0) in component "10_Modulo_cannone_reale_PCB_solenoide_canna"
sketch "Schizzo6 (8)" plane through (0, 0, 85.5) normal (0, 0, 1) x (1, 0, 0) in component "10_Modulo_cannone_reale_PCB_solenoide_canna"
  line L0 (-10, 2.5) -> (10, 2.5)
  line L1 (10, 2.5) -> (10, 27.5)
  line L2 (10, 27.5) -> (-10, 27.5)
  line L3 (-10, 27.5) -> (-10, 2.5)
extrude "Estrusione_Appoggio_solenoide_su_PCB" add sketch "Schizzo6 (8)" along normal blind 1 separate body makes body 21 in component "10_Modulo_cannone_reale_PCB_solenoide_canna"
ref_plane "Piano di lavoro3" through (0, 2.5, 0) normal (0, 1, 0) x (0, 0, 1) in component "10_Modulo_cannone_reale_PCB_solenoide_canna"
sketch "Schizzo7 (8)" plane through (0, 2.5, 0) normal (0, 1, 0) x (1, 0, 0) in component "10_Modulo_cannone_reale_PCB_solenoide_canna"
  circle A0 centre (0, -96.5) radius 10
extrude "Estrusione_Corpo_solenoide_riferimento" add sketch "Schizzo7 (8)" along normal blind 25 separate body makes body 22 in component "10_Modulo_cannone_reale_PCB_solenoide_canna"
ref_plane "Piano di lavoro4" through (0, 2.5, 0) normal (0, 1, 0) x (0, 0, 1) in component "10_Modulo_cannone_reale_PCB_solenoide_canna"
sketch "Schizzo8 (8)" plane through (0, 2.5, 0) normal (0, 1, 0) x (1, 0, 0) in component "10_Modulo_cannone_reale_PCB_solenoide_canna"
  circle A0 centre (0, -96.5) radius 5
extrude "Passaggio_canna_nel_solenoide" cut sketch "Schizzo8 (8)" along normal blind 25 bodies 22 in component "10_Modulo_cannone_reale_PCB_solenoide_canna"
ref_plane "Piano di lavoro5" through (0, 27.5, 0) normal (0, 1, 0) x (0, 0, 1) in component "10_Modulo_cannone_reale_PCB_solenoide_canna"
sketch "Schizzo9 (8)" plane through (0, 27.5, 0) normal (0, 1, 0) x (1, 0, 0) in component "10_Modulo_cannone_reale_PCB_solenoide_canna"
  circle A0 centre (0, -96.5) radius 5
extrude "Estrusione_Canna_tubolare_esterna" add sketch "Schizzo9 (8)" along normal blind 46 separate body makes body 23 in component "10_Modulo_cannone_reale_PCB_solenoide_canna"
ref_plane "Piano di lavoro6" through (0, 27.5, 0) normal (0, 1, 0) x (0, 0, 1) in component "10_Modulo_cannone_reale_PCB_solenoide_canna"
sketch "Schizzo10 (8)" plane through (0, 27.5, 0) normal (0, 1, 0) x (1, 0, 0) in component "10_Modulo_cannone_reale_PCB_solenoide_canna"
  circle A0 centre (0, -96.5) radius 4
extrude "Foro_interno_canna_tubolare" cut sketch "Schizzo10 (8)" along normal blind 46 bodies 23 in component "10_Modulo_cannone_reale_PCB_solenoide_canna"
ref_plane "Piano di lavoro1" through (0, -38, 0) normal (0, 1, 0) x (0, 0, 1) in component "11_Guscio_fisso_posteriore_torretta_removibile"
sketch "Schizzo1 (20)" plane through (0, -38, 0) normal (0, 1, 0) x (1, 0, 0) in component "11_Guscio_fisso_posteriore_torretta_removibile"
  line L0 (-43, -49.5) -> (43, -49.5)
  line L1 (43, -49.5) -> (43, -102.5)
  line L2 (43, -102.5) -> (-43, -102.5)
  line L3 (-43, -102.5) -> (-43, -49.5)
extrude "Estrusione_Parete_posteriore_guscio_torretta" add sketch "Schizzo1 (20)" along normal blind 2.5 separate body makes body 24 in component "11_Guscio_fisso_posteriore_torretta_removibile"
ref_plane "Piano di lavoro2" through (-43, 0, 0) normal (1, 0, 0) x (0, 1, 0) in component "11_Guscio_fisso_posteriore_torretta_removibile"
sketch "Schizzo2 (18)" plane through (-43, 0, 0) normal (1, 0, 0) x (0, 0, -1) in component "11_Guscio_fisso_posteriore_torretta_removibile"
  line L0 (-49.5, -38) -> (-102.5, -38)
  line L1 (-102.5, -38) -> (-102.5, -27.8)
  line L2 (-102.5, -27.8) -> (-49.5, -27.8)
  line L3 (-49.5, -27.8) -> (-49.5, -38)
extrude "Estrusione_Fianco_cofano_Sinistra" add sketch "Schizzo2 (18)" along normal blind 2.5 bodies 24 in component "11_Guscio_fisso_posteriore_torretta_removibile"
ref_plane "Piano di lavoro3" through (40.5, 0, 0) normal (1, 0, 0) x (0, 1, 0) in component "11_Guscio_fisso_posteriore_torretta_removibile"
sketch "Schizzo3 (16)" plane through (40.5, 0, 0) normal (1, 0, 0) x (0, 0, -1) in component "11_Guscio_fisso_posteriore_torretta_removibile"
  line L0 (-49.5, -38) -> (-102.5, -38)
  line L1 (-102.5, -38) -> (-102.5, -27.8)
  line L2 (-102.5, -27.8) -> (-49.5, -27.8)
  line L3 (-49.5, -27.8) -> (-49.5, -38)
extrude "Estrusione_Fianco_cofano_Destra" add sketch "Schizzo3 (16)" along normal blind 2.5 bodies 24 in component "11_Guscio_fisso_posteriore_torretta_removibile"
ref_plane "Piano di lavoro4" through (0, 0, 100) normal (0, 0, 1) x (1, 0, 0) in component "11_Guscio_fisso_posteriore_torretta_removibile"
sketch "Schizzo4 (16)" plane through (0, 0, 100) normal (0, 0, 1) x (1, 0, 0) in component "11_Guscio_fisso_posteriore_torretta_removibile"
  line L0 (-43, -38) -> (43, -38)
  line L1 (43, -38) -> (43, -27.8)
  line L2 (43, -27.8) -> (-43, -27.8)
  line L3 (-43, -27.8) -> (-43, -38)
extrude "Estrusione_Tetto_cofano_posteriore" add sketch "Schizzo4 (16)" along normal blind 2.5 bodies 24 in component "11_Guscio_fisso_posteriore_torretta_removibile"
ref_plane "Piano di lavoro5" through (-43, 0, 0) normal (1, 0, 0) x (0, 1, 0) in component "11_Guscio_fisso_posteriore_torretta_removibile"
sketch "Schizzo5 (9)" plane through (-43, 0, 0) normal (1, 0, 0) x (0, 0, -1) in component "11_Guscio_fisso_posteriore_torretta_removibile"
  circle A0 centre (-54.5, -30.3) radius 1.35
extrude "Foro_M2_5_cofano_Sinistra_01" cut sketch "Schizzo5 (9)" along normal blind 2.5 bodies 24 in component "11_Guscio_fisso_posteriore_torretta_removibile"
ref_plane "Piano di lavoro23" through (-40, 0, 0) normal (1, 0, 0) x (0, 1, 0) in component "04_Torretta_parte_fissa_azimut"
sketch "Schizzo37 (2)" plane through (-40, 0, 0) normal (1, 0, 0) x (0, 0, -1) in component "04_Torretta_parte_fissa_azimut"
  circle A0 centre (-54.5, -30.3) radius 1.1
extrude "Preforo_M2_5_cofano_telaio_Sinistra_01" cut sketch "Schizzo37 (2)" along normal blind 4 bodies 12 in component "04_Torretta_parte_fissa_azimut"
ref_plane "Piano di lavoro6" through (-43, 0, 0) normal (1, 0, 0) x (0, 1, 0) in component "11_Guscio_fisso_posteriore_torretta_removibile"
sketch "Schizzo6 (9)" plane through (-43, 0, 0) normal (1, 0, 0) x (0, 0, -1) in component "11_Guscio_fisso_posteriore_torretta_removibile"
  circle A0 centre (-94.5, -30.3) radius 1.35
extrude "Foro_M2_5_cofano_Sinistra_02" cut sketch "Schizzo6 (9)" along normal blind 2.5 bodies 24 in component "11_Guscio_fisso_posteriore_torretta_removibile"
ref_plane "Piano di lavoro24" through (-40, 0, 0) normal (1, 0, 0) x (0, 1, 0) in component "04_Torretta_parte_fissa_azimut"
sketch "Schizzo38 (2)" plane through (-40, 0, 0) normal (1, 0, 0) x (0, 0, -1) in component "04_Torretta_parte_fissa_azimut"
  circle A0 centre (-94.5, -30.3) radius 1.1
extrude "Preforo_M2_5_cofano_telaio_Sinistra_02" cut sketch "Schizzo38 (2)" along normal blind 4 bodies 12 in component "04_Torretta_parte_fissa_azimut"
ref_plane "Piano di lavoro7" through (40.5, 0, 0) normal (1, 0, 0) x (0, 1, 0) in component "11_Guscio_fisso_posteriore_torretta_removibile"
sketch "Schizzo7 (9)" plane through (40.5, 0, 0) normal (1, 0, 0) x (0, 0, -1) in component "11_Guscio_fisso_posteriore_torretta_removibile"
  circle A0 centre (-54.5, -30.3) radius 1.35
extrude "Foro_M2_5_cofano_Destra_01" cut sketch "Schizzo7 (9)" along normal blind 2.5 bodies 24 in component "11_Guscio_fisso_posteriore_torretta_removibile"
ref_plane "Piano di lavoro25" through (36, 0, 0) normal (1, 0, 0) x (0, 1, 0) in component "04_Torretta_parte_fissa_azimut"
sketch "Schizzo39 (2)" plane through (36, 0, 0) normal (1, 0, 0) x (0, 0, -1) in component "04_Torretta_parte_fissa_azimut"
  circle A0 centre (-54.5, -30.3) radius 1.1
extrude "Preforo_M2_5_cofano_telaio_Destra_01" cut sketch "Schizzo39 (2)" along normal blind 4 bodies 12 in component "04_Torretta_parte_fissa_azimut"
ref_plane "Piano di lavoro8" through (40.5, 0, 0) normal (1, 0, 0) x (0, 1, 0) in component "11_Guscio_fisso_posteriore_torretta_removibile"
sketch "Schizzo8 (9)" plane through (40.5, 0, 0) normal (1, 0, 0) x (0, 0, -1) in component "11_Guscio_fisso_posteriore_torretta_removibile"
  circle A0 centre (-94.5, -30.3) radius 1.35
extrude "Foro_M2_5_cofano_Destra_02" cut sketch "Schizzo8 (9)" along normal blind 2.5 bodies 24 in component "11_Guscio_fisso_posteriore_torretta_removibile"
ref_plane "Piano di lavoro26" through (36, 0, 0) normal (1, 0, 0) x (0, 1, 0) in component "04_Torretta_parte_fissa_azimut"
sketch "Schizzo40 (2)" plane through (36, 0, 0) normal (1, 0, 0) x (0, 0, -1) in component "04_Torretta_parte_fissa_azimut"
  circle A0 centre (-94.5, -30.3) radius 1.1
extrude "Preforo_M2_5_cofano_telaio_Destra_02" cut sketch "Schizzo40 (2)" along normal blind 4 bodies 12 in component "04_Torretta_parte_fissa_azimut"
ref_plane "Piano di lavoro1" through (-69.5, 0, 0) normal (1, 0, 0) x (0, 1, 0) in component "12_Carter_SG90_Sinistro_removibile"
sketch "Schizzo1 (21)" plane through (-69.5, 0, 0) normal (1, 0, 0) x (0, 0, -1) in component "12_Carter_SG90_Sinistro_removibile"
  line L0 (-71.9, -27.8) -> (-93.6, -27.8)
  line L1 (-93.6, -27.8) -> (-93.6, 16.5)
  line L2 (-93.6, 16.5) -> (-71.9, 16.5)
  line L3 (-71.9, 16.5) -> (-71.9, -27.8)
extrude "Estrusione_Parete_esterna_carter_Sinistro" add sketch "Schizzo1 (21)" along normal blind 2.5 separate body makes body 25 in component "12_Carter_SG90_Sinistro_removibile"
ref_plane "Piano di lavoro2" through (0, -27.8, 0) normal (0, 1, 0) x (0, 0, 1) in component "12_Carter_SG90_Sinistro_removibile"
sketch "Schizzo2 (19)" plane through (0, -27.8, 0) normal (0, 1, 0) x (1, 0, 0) in component "12_Carter_SG90_Sinistro_removibile"
  line L0 (-69.5, -71.9) -> (-40.5, -71.9)
  line L1 (-40.5, -71.9) -> (-40.5, -93.6)
  line L2 (-40.5, -93.6) -> (-69.5, -93.6)
  line L3 (-69.5, -93.6) -> (-69.5, -71.9)
extrude "Estrusione_Parete_Posteriore_carter_Sinistro" add sketch "Schizzo2 (19)" along normal blind 2.5 bodies 25 in component "12_Carter_SG90_Sinistro_removibile"
ref_plane "Piano di lavoro3" through (0, 14, 0) normal (0, 1, 0) x (0, 0, 1) in component "12_Carter_SG90_Sinistro_removibile"